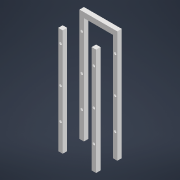
# Autodesk Inventor part: Sustentação Trilhos fixos
Saved by Autodesk Inventor 2022 (Build 260153000, 153)
## iProperties
Created: 2023-05-11
Part Number: Sustentação Trilhos fixos
Material: Genérico
Document SubType Name: Modeling
Designer: jpjoa
Density: 1 g/cm^3
Appearance: Padrão
Author: jpjoa
Autodesk Inventor part; units mm, degrees
ref_plane "YZ Plane" through (0, 0, 0) normal (1, 0, 0) x (0, 1, 0)
ref_plane "XZ Plane" through (0, 0, 0) normal (0, 1, 0) x (-1, 0, 0)
ref_plane "XY Plane" through (0, 0, 0) normal (0, 0, 1) x (1, 0, 0)
sketch "Esboço1" plane through (0, 0, 0) normal (0, 1, 0) x (-1, 0, 0)
  line L0 (0, 0) -> (0, -5.4)
  line L1 (0, -5.4) -> (5.4, -5.4)
  line L2 (5.4, -5.4) -> (5.4, 0)
  line L3 (5.4, 0) -> (0, 0)
  line L4 (40.622, 0) -> (40.622, -5.4)
  line L5 (40.622, -5.4) -> (46.022, -5.4)
  line L6 (46.022, -5.4) -> (46.022, 0)
  line L7 (46.022, 0) -> (40.622, 0)
  line L8 (40.622, 0) -> (5.4, 0)
  line L9 (5.4, -5.4) -> (40.622, -5.4)
  point P0 (0, -2.7)
  point P1 (5.4, -2.7)
  point P2 (40.622, -2.7)
  point P3 (46.022, -2.7)
  point P4 (43.322, -5.4)
  point P5 (2.7, -5.4)
  point P6 (43.322, 0)
  point P7 (2.7, 0)
  point P8 (0, 0)
  dimension "d29" = 35.222
  dimension "d30" = 5.4
  constraints: 20 end point, 8 midpoint, 6 perpendicular, 2 coincident, 2 equal length, 2 horizontal alignment, 2 vertical, 1 collinear, 1 horizontal
  measures "d29" distance between parallel lines of L2 L4
  measures "d30" distance of L4.end L5.end
extrude "Extrusão1" add sketch "Esboço1" against normal blind 130 contours L3 L2 L1 L0 | L7 L6 L5 L4
extrude "Extrusão4" add sketch "Esboço1" along normal blind 5.4
sketch "Esboço5" plane through (-40.622, 0, 0) normal (0, 0, 1) x (1, 0, 0)
  circle A0 centre (37.922, -56.6141) radius 1.5
  circle A1 centre (37.922, -45.6701) radius 1.5
  circle A2 centre (37.922, -36.5809) radius 1.5
  circle A3 centre (-2.7, -55.1141) radius 1.5
  circle A4 centre (-2.7, -45.6701) radius 1.5
  circle A5 centre (-2.7, -32.1291) radius 1.5
  line L0 (40.622, -130) -> (35.222, -130) projected
  line L1 (0, -130) -> (-5.4, -130) projected
  point P0 (40.622, 0)
  point P1 (37.922, -130)
  point P2 (-2.7, -130)
  dimension "d33" = 3
  dimension "d34" = 3
  dimension "d36" = 3
  dimension "d38" = 3
  dimension "d40" = 3
  dimension "d42" = 3
  constraints: 6 centre point, 6 vertical alignment, 2 midpoint
  measures "d33" diameter of A0
  measures "d34" diameter of A1
  measures "d36" diameter of A2
  measures "d38" diameter of A3
  measures "d40" diameter of A4
  measures "d42" diameter of A5
equation "\"d29\" = Largura_trilhos"
equation "\"d33\" = Parafuso"
equation "\"d34\" = d35"
equation "\"d36\" = d37"
equation "\"d38\" = d39"
equation "\"d40\" = d41"
equation "\"d42\" = d43"
equation "\"Largura_trilhos\" = 35.222"
equation "\"Parafuso\" = 3"
equation "\"d11\" = 3"
equation "\"d13\" = 3"
equation "\"d15\" = 3"
equation "\"d17\" = 3"
equation "\"d19\" = 3"
equation "\"d35\" = 3"
equation "\"d37\" = 3"
equation "\"d39\" = 3"
equation "\"d41\" = 3"
equation "\"d43\" = 3"
